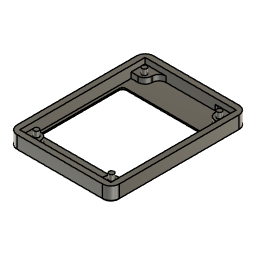
TFT Display Holder V3 v3 (Autodesk Fusion 360 design; units mm, degrees)
Autodesk Fusion 360 part; units mm, degrees
note: some values were not read from the file. Chosen so that the rebuilt part matches the saved one: which face or edge a step refers to. Set by a fixed rule: which sketch regions a step uses.
sketch "Sketch1" plane through (0, 0, 0) normal (0, 0, 1) x (1, 0, 0)
  line L0 (3, 0) -> (33.5, 0)
  line L1 (36.5, 3) -> (36.5, 45.7)
  line L2 (33.5, 48.7) -> (3, 48.7)
  line L3 (0, 45.7) -> (0, 3)
  line L4 (2, 2) -> (34.5, 2)
  line L5 (34.5, 2) -> (34.5, 46.7)
  line L6 (34.5, 46.7) -> (2, 46.7)
  line L7 (2, 46.7) -> (2, 2)
  circle A0 centre (4.85, 5.1) radius 0.8998
  circle A1 centre (31.65, 5.1) radius 0.9
  circle A2 centre (31.65, 43.6) radius 0.9002
  circle A3 centre (4.85, 43.6) radius 0.8999
  line L8 (4, 37.7) -> (32.5, 37.7)
  line L9 (33.5, 36.7) -> (33.5, 9)
  line L10 (32.5, 8) -> (4, 8)
  line L11 (3, 9) -> (3, 36.7)
  line L12 (2, 46.7) -> (7, 46.7)
  line L13 (7, 46.7) -> (7, 44.2)
  line L14 (4.5, 41.7) -> (2, 41.7)
  line L15 (2, 41.7) -> (2, 46.7)
  line L16 (34.5, 46.7) -> (29.5, 46.7)
  line L17 (29.5, 46.7) -> (29.5, 44.2)
  line L18 (32, 41.7) -> (34.5, 41.7)
  line L19 (34.5, 41.7) -> (34.5, 46.7)
  line L20 (34.5, 2) -> (29.5, 2)
  line L21 (29.5, 2) -> (29.5, 4.5)
  line L22 (32, 7) -> (34.5, 7)
  line L23 (34.5, 7) -> (34.5, 2)
  line L24 (2, 2) -> (7, 2)
  line L25 (7, 2) -> (7, 4.5)
  line L26 (4.5, 7) -> (2, 7)
  line L27 (2, 7) -> (2, 2)
  arc A4 (33.5, 36.7) -> (32.5, 37.7) centre (32.5, 36.7) ccw
  arc A5 (4, 37.7) -> (3, 36.7) centre (4, 36.7) ccw
  arc A6 (3, 9) -> (4, 8) centre (4, 9) ccw
  arc A7 (32.5, 8) -> (33.5, 9) centre (32.5, 9) ccw
  arc A8 (33.5, 0) -> (36.5, 3) centre (33.5, 3) ccw
  arc A9 (0, 3) -> (3, 0) centre (3, 3) ccw
  arc A10 (3, 48.7) -> (0, 45.7) centre (3, 45.7) ccw
  arc A11 (36.5, 45.7) -> (33.5, 48.7) centre (33.5, 45.7) ccw
  arc A12 (32, 7) -> (29.5, 4.5) centre (32, 4.5) ccw
  arc A13 (7, 4.5) -> (4.5, 7) centre (4.5, 4.5) ccw
  arc A14 (29.5, 44.2) -> (32, 41.7) centre (32, 44.2) ccw
  arc A15 (4.5, 41.7) -> (7, 44.2) centre (4.5, 44.2) ccw
  dimension "d23" = 1
  dimension "d24" = 3
  dimension "d25" = 2.5
  constraint horizontal L0
  constraint vertical L1
  constraint horizontal L2
  constraint vertical L3
  constraint horizontal L4
  constraint vertical L5
  constraint horizontal L6
  constraint vertical L7
  constraint horizontal L8
  constraint vertical L9
  constraint horizontal L10
  constraint vertical L11
  constraint horizontal L12
  constraint vertical L13
  constraint horizontal L14
  constraint vertical L15
  constraint horizontal L16
  constraint vertical L17
  constraint horizontal L18
  constraint vertical L19
  constraint horizontal L20
  constraint vertical L21
  constraint horizontal L22
  constraint vertical L23
  constraint horizontal L24
  constraint vertical L25
  constraint horizontal L26
  constraint vertical L27
  constraint tangent L8 A4
  constraint tangent L9 A4
  constraint tangent L8 A5
  constraint tangent L11 A5
  constraint equal A4 A5
  constraint tangent L10 A6
  constraint tangent L11 A6
  constraint equal A4 A6
  constraint tangent L9 A7
  constraint tangent L10 A7
  constraint equal A4 A7
  constraint tangent L0 A8
  constraint tangent L1 A8
  constraint tangent L0 A9
  constraint tangent L3 A9
  constraint equal A8 A9
  constraint tangent L2 A10
  constraint tangent L3 A10
  constraint equal A8 A10
  constraint tangent L1 A11
  constraint tangent L2 A11
  constraint equal A8 A11
  constraint tangent L21 A12
  constraint tangent L22 A12
  constraint tangent L25 A13
  constraint tangent L26 A13
  constraint equal A12 A13
  constraint tangent L17 A14
  constraint tangent L18 A14
  constraint equal A12 A14
  constraint tangent L13 A15
  constraint tangent L14 A15
  constraint equal A12 A15
  measures "d23" radius of A4
  measures "d24" radius of A8
  measures "d25" radius of A12
extrude "Extrude1" add sketch "Sketch1" along normal blind 1 contours L0 L1 L2 L3 A8 A9 A10 A11 | L4 L7 L24 L25 L26 L27 A13 | L4 L5 L6 L7 L13 L14 L17 L18 L21 L22 L25 L26 A12 A13 A14 A15 | L4 L5 L20 L21 L22 L23 A12 | L6 L7 L12 L13 L14 L15 A15 | L5 L6 L16 L17 L18 L19 A14 | A0 | A1 | A2 | A3
extrude "Extrude2" cut sketch "Sketch1" along normal blind 4 contours L4 L7 L24 L25 L26 L27 A13 | L4 L5 L20 L21 L22 L23 A12 | L6 L7 L12 L13 L14 L15 A15 | L5 L6 L16 L17 L18 L19 A14 | A0 | A1 | A2 | A3
extrude "Extrude3" add sketch "Sketch1" along normal blind 4 contours L4 L7 L24 L25 L26 L27 A13 | L4 L5 L20 L21 L22 L23 A12 | L6 L7 L12 L13 L14 L15 A15 | L5 L6 L16 L17 L18 L19 A14 | A0 | A1 | A2 | A3
extrude "Extrude4" cut sketch "Sketch1" along normal blind 5 contours A0 | A1 | A2 | A3
extrude "Extrude5" add sketch "Sketch1" along normal blind 6 contours A0 | A1 | A2 | A3
extrude "Extrude6" cut sketch "Sketch1" along normal blind 4 contours L0 L1 L2 L3 A8 A9 A10 A11
extrude "Extrude7" add sketch "Sketch1" along normal blind 6 contours L0 L1 L2 L3 A8 A9 A10 A11
extrude "Extrude8" cut 4 faces at (4.5943, 2.7343, 4) (31.9058, 2.7342, 4) (4.5943, 45.9658, 4) (31.9058, 45.9659, 4) along direction (0, 0, -1) blind 1
extrude "Extrude9" cut 5 faces at (31.7168, 43.3075, 6) (35.1667, 31.4667, 6) (4.8534, 43.5553, 6) (5.1663, 4.8815, 6) (31.3602, 5.3598, 6) along direction (0, 0, -1) blind 1
fillet "Fillet1" [no effect]
fillet "Fillet2" radius 2.5 8 edges at (7, 2, 2) (29.5, 2, 2) (29.5, 46.7, 2) (7, 46.7, 2) (7, 3.25, 1) (7, 45.45, 1) (29.5, 45.45, 1) (29.5, 3.25, 1)
chamfer "Chamfer1" distance 0.5 angle 45 8 edges at (18.25, 0, 0) (35.6213, 0.8787, 0) (36.5, 24.35, 0) (35.6213, 47.8213, 0) (18.25, 48.7, 0) (0.8787, 47.8213, 0) (0, 24.35, 0) (0.8787, 0.8787, 0)
chamfer "Chamfer2" distance 0.5 angle 45 8 edges at (18.25, 37.7, 0) (33.2071, 37.4071, 0) (33.5, 22.85, 0) (33.2071, 8.2929, 0) (18.25, 8, 0) (3.2929, 8.2929, 0) (3, 22.85, 0) (3.2929, 37.4071, 0)
